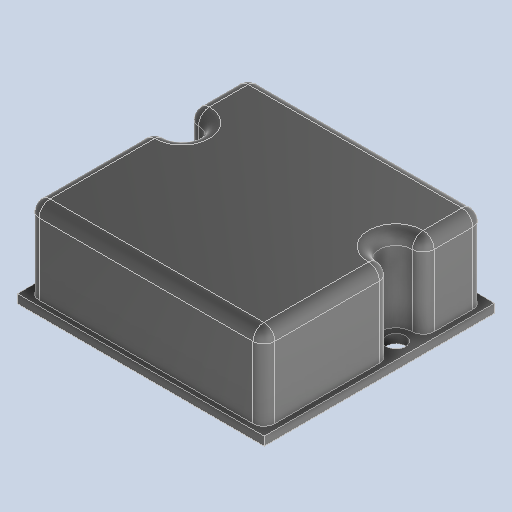
# Autodesk Inventor part: AKI.DAC-U2704 REV.C
Saved by Autodesk Inventor 2024.2 (Build 282272000, 272)
## iProperties
Created: 2024-02-01
Part Number: AKI.DAC-U2704 REV.C
Material: Acetal Resin, Black
Document SubType Name: Modeling
Designer: Masato Kubotera
Density: 1.425 g/cm^3
Appearance: Smooth - Black
Author: Masato Kubotera
Autodesk Inventor part; units mm, degrees
ref_plane "YZ Plane" through (0, 0, 0) normal (1, 0, 0) x (0, 1, 0)
ref_plane "XZ Plane" through (0, 0, 0) normal (0, 1, 0) x (-1, 0, 0)
ref_plane "XY Plane" through (0, 0, 0) normal (0, 0, 1) x (1, 0, 0)
sketch "Sketch1" plane through (0, 0, 0) normal (0, 0, 1) x (1, 0, 0)
  line L0 (-21, 22.5) -> (21, 22.5)
  line L1 (21, 22.5) -> (21, -22.5)
  line L2 (21, -22.5) -> (-21, -22.5)
  line L3 (-21, -22.5) -> (-21, 22.5)
  line L4 (-21, 22.5) -> (21, -22.5) construction
  line L5 (21, 22.5) -> (-21, -22.5) construction
  line L6 (-6, 19.5) -> (-6, -19.5) construction
  line L7 (-21, 0) -> (21, 0) construction
  arc A0 (-8.2361, 21.5) -> (-3.7639, 21.5) centre (-6, 19.5) ccw
  line L8 (20.0667, -21.5) -> (-20.0667, -21.5)
  line L9 (-20.0667, -21.5) -> (-20.0667, 21.5)
  line L10 (-20.0667, 21.5) -> (20.0667, 21.5)
  line L11 (20.0667, 21.5) -> (20.0667, -21.5)
  line L12 (20.0667, -21.5) -> (-20.0667, 21.5) construction
  line L13 (-20.0667, -21.5) -> (20.0667, 21.5) construction
  arc A1 (-3.7639, -21.5) -> (-8.2361, -21.5) centre (-6, -19.5) ccw
  point P0 (0, 0)
  point P1 (-8.2361, -21.5)
  point P2 (-3.7639, -21.5)
  dimension "d0" = 42
  dimension "d1" = 45
  dimension "d2" = 15
  dimension "d3" = 39
  dimension "d6" = 1
  dimension "d7" = 6
  constraints: 28 end point, 6 midpoint, 4 parallel, 4 point on circle, 4 symmetric about line, 3 coincident, 3 point on line, 2 centre point, 2 horizontal, 2 perpendicular, 1 vertical, 1 other
  measures "d0" distance of L1.end L2.end
  measures "d1" distance of L0.end L1.end
  measures "d2" distance between parallel lines of L3 L6
  measures "d3" distance of L6.start L6.end
  measures "d6" distance between parallel lines of L10 L0
  measures "d7" diameter of A0
extrude "Extrusion1" add sketch "Sketch1" against normal blind 1.6 contours L0 L1 L2 L3 | L10 A0 | A0 L10 L11 L8 A1 L9 | A1 L8
extrude "Extrusion2" add sketch "Sketch1" along normal blind 15 contours A0 L10 L11 L8 A1 L9
fillet "Fillet1" radius 2 16 edges at (-3.7639, 21.5, 7.5) (-8.2361, 21.5, 7.5) (-3.7639, -21.5, 7.5) (-8.2361, -21.5, 7.5) (-20.0667, 21.5, 7.5) (-20.0667, -21.5, 7.5) (20.0667, -21.5, 7.5) (20.0667, 21.5, 7.5) (20.0667, 0, 15) (8.1514, 21.5, 15) (-14.1514, 21.5, 15) (-6, 16.5, 15) (-20.0667, 0, 15) (-14.1514, -21.5, 15) (-6, -16.5, 15) (8.1514, -21.5, 15)
hole "Hole1" at (-6, 19.5, 0) at (-6, -19.5, 0) direction (0, 0, -1) diameter 3.5 end through all
body "Solid1"
